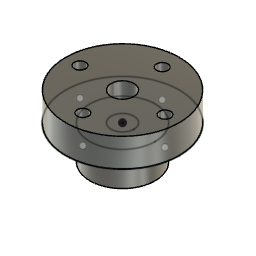
gear motor 1 (Autodesk Fusion 360 design; units mm, degrees)
Autodesk Fusion 360 part; units mm, degrees
note: some values were not read from the file. Set by a fixed rule: the direction of a hole.
sketch "Sketch1" plane through (0, 0, 0) normal (0, 0, 1) x (1, 0, 0)
  circle A0 centre (0, 0) radius 20
  circle A1 centre (0, 0) radius 4
  circle A2 centre (0, 0) radius 11.5
  point P0 (-15, 0)
  point P1 (15, 0)
  point P2 (0, 14)
  point P3 (0, -14)
  dimension "d1" = 40
  dimension "d2" = 8
  dimension "d3" = 15
  dimension "d4" = 15
  dimension "d5" = 14
  dimension "d6" = 14
  dimension "d7" = 23
  constraint coincident A0.centre A1.centre
  constraint concentric A0 A1
  measures "d1" diameter of A0
  measures "d2" diameter of A1
  measures "d3" distance of A0.centre P0
  measures "d4" distance of A0.centre P1
  measures "d5" distance of A0.centre P2
  measures "d6" distance of A0.centre P3
  measures "d7" diameter of A2
extrude "Extrude1" add sketch "Sketch1" along normal blind 10 contours A0 | A2
extrude "Extrude2" add sketch "Sketch1" against normal blind 12 contours A2
hole "Hole1" at (0, 14, 0) at (15, 0, 0) at (0, -14, 0) at (-15, 0, 0) direction (0, 0, 1) diameter 4 depth 20 tip angle 118
ref_plane "WorkPlane1" through (8.1317, 8.1317, -4.9786) normal (0.707107, 0.707107, 0) x (-0.707107, 0.707107, 0)
hole "Hole2" at (7.9968, 8.2666, -5.7724) direction (-0.707107, -0.707107, 0) diameter 4 depth 12 tip angle 118
